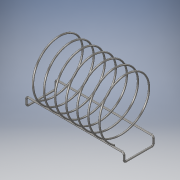
# Autodesk Inventor part: Toast Rack
Saved by Autodesk Inventor 2018 (Build 220112000, 112)
## iProperties
Created: 2017-09-21
Part Number: Toast Rack
Material: Stainless Steel
Document SubType Name: Modeling
Designer: kurtis
Density: 8 g/cm^3
Appearance: Semi-Polished
Author: kurtis
Autodesk Inventor part; units mm, degrees
ref_plane "YZ Plane" through (0, 0, 0) normal (1, 0, 0) x (0, 1, 0)
ref_plane "Work Plane1" through (129.4372, -11.3801, 19.1698) normal (0, 0, -1) x (-1, 0, 0)
sketch "Sketch4" plane through (129.4372, -11.3801, 19.1698) normal (0, 0, -1) x (-1, 0, 0)
  circle A0 centre (0, 0) radius 1.5
  point P0 (129.4372, 11.3801)
  dimension "d10" = 3
  constraints: 1 centre point
  measures "d10" diameter of A0
sketch3d "3D Sketch1"
  line L0 (-46.5628, -11.3801, 42.6698) -> (-46.5628, -11.3801, -4.3302)
  arc A0 (-46.5628, -11.3801, -4.3302) -> (-46.5628, -8.3801, -7.3302) centre (-46.5628, -8.3801, -4.3302) ccw
  line L1 (-46.5628, -8.3801, -7.3302) -> (-46.5628, 0.6199, -7.3302)
  arc A1 (-46.5628, 0.6199, -7.3302) -> (-43.5628, 3.6199, -7.3302) centre (-43.5628, 0.6199, -7.3302) ccw
  line L2 (-43.5628, 3.6199, -7.3302) -> (126.4372, 3.6199, -7.3302)
  arc A2 (126.4372, 3.6199, -7.3302) -> (129.4372, 0.6199, -7.3302) centre (126.4372, 0.6199, -7.3302) ccw
  line L3 (129.4372, 0.6199, -7.3302) -> (129.4372, -8.3801, -7.3302)
  arc A3 (129.4372, -8.3801, -7.3302) -> (129.4372, -11.3801, -4.3302) centre (129.4372, -8.3801, -4.3302) ccw
  line L4 (129.4372, -11.3801, -4.3302) -> (129.4372, -11.3801, 42.6698)
  arc A4 (129.4372, -11.3801, 42.6698) -> (129.4372, -8.3801, 45.6698) centre (129.4372, -8.3801, 42.6698) ccw
  line L5 (129.4372, -8.3801, 45.6698) -> (129.4372, 0.6199, 45.6698)
  arc A5 (129.4372, 0.6199, 45.6698) -> (126.4372, 3.6199, 45.6698) centre (126.4372, 0.6199, 45.6698) ccw
  line L6 (126.4372, 3.6199, 45.6698) -> (-43.5628, 3.6199, 45.6698)
  arc A6 (-43.5628, 3.6199, 45.6698) -> (-46.5628, 0.6199, 45.6698) centre (-43.5628, 0.6199, 45.6698) ccw
  line L7 (-46.5628, 0.6199, 45.6698) -> (-46.5628, -8.3801, 45.6698)
  arc A7 (-46.5628, -8.3801, 45.6698) -> (-46.5628, -11.3801, 42.6698) centre (-46.5628, -8.3801, 42.6698) ccw
  dimension "d0" = 53
  dimension "d1" = 15
  dimension "d2" = 176
  dimension "d3" = 15
  dimension "d4" = 53
  dimension "d5" = 15
  dimension "d6" = 176
  dimension "d11" = 3
  dimension "d12" = 3
  dimension "d13" = 3
  dimension "d14" = 3
  dimension "d15" = 3
  dimension "d16" = 3
  dimension "d17" = 3
  dimension "d18" = 3
sweep "Sweep1" add profiles "Sketch4" path "3D Sketch1"
ref_plane "Work Plane3" through (126.4372, 0.6199, 45.6698) normal (0, 0, 1) x (1, 0, 0)
sketch "Sketch6" plane through (126.4372, 0.6199, 45.6698) normal (0, 0, 1) x (1, 0, 0)
  line L0 (0, 0) -> (3, 0) construction
  line L1 (1.5, 0) -> (4.5, 0) construction
  line L2 (3, 0) -> (-15, 0) construction
  line L3 (-15, 0) -> (-15, 6) construction
  circle A0 centre (-15, 6) radius 1.5
  point P0 (-126.4372, -0.6199)
  dimension "d27" = 18
  dimension "d28" = 6
  dimension "d29" = 3
  constraints: 6 end point, 1 centre point, 1 coincident, 1 midpoint, 1 point on line, 1 vertical
  measures "d27" distance of L0.end L2.end
  measures "d28" distance of L2.end L3.end
  measures "d29" diameter of A0
ref_plane "Work Plane7" through (126.4372, 0.6199, 19.1698) normal (0, 0, -1) x (-1, 0, 0)
ref_plane "Work Plane6" through (126.4372, 0.6199, -7.3302) normal (0, 0, -1) x (-1, 0, 0)
sketch "Sketch8" plane through (126.4372, 0.6199, 19.1698) normal (0, 0, -1) x (-1, 0, 0)
  circle A0 centre (-3, -12) radius 1.5 construction
  line L0 (-3, -12) -> (-3, 48) construction
  line L1 (-3, 48) -> (173, 48)
  point P0 (126.4372, -0.6199)
  dimension "d33" = 60
  dimension "d34" = 176
  constraints: 4 end point, 1 perpendicular, 1 vertical
  measures "d33" distance of L0.start L0.end
  measures "d34" distance of L0.end L1.end
coil "Coil1" sketch "Sketch6" operation add axis through (129.4372, 48.6199, 19.1698) along (-1, 0, 0) pitch 20 turns 7 hand right
equation "\"d12\" = d11"
equation "\"d13\" = d11"
equation "\"d14\" = d11"
equation "\"d16\" = d15"
equation "\"d17\" = d15"
equation "\"d18\" = d15"
body "Solid1"
